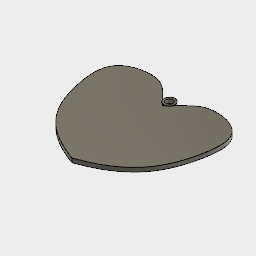
FPROJ_11_LIUYH (Autodesk Fusion 360 design; units mm, degrees)
Autodesk Fusion 360 part; units mm, degrees
sketch "草图1" plane through (0, 0, 0) normal (0, 1, 0) x (1, 0, 0)
  spline S0 degree 5 poles (0, 0) (-0.5793, 0.5821) (-1.7157, 1.7269) (-3.3538, 3.3854) (-5.4045, 5.4793) (-7.7689, 7.8927) (-10.0073, 10.0799) (-12.2674, 11.9974) (-14.7989, 13.5743) (-17.8484, 14.7231) (-21.5675, 15.3505) (-25.8885, 15.3683) (-30.5109, 14.703) (-35.0251, 13.3026) (-39.0061, 11.1441) (-42.1086, 8.2405) (-44.187, 4.6516) (-45.2856, 0.4771) (-45.5576, -4.1594) (-45.2061, -9.1233) (-44.4201, -14.2831) (-43.3041, -19.5247) (-41.886, -24.7523) (-40.1407, -29.8862) (-38.0071, -34.8616) (-35.4076, -39.6274) (-32.2667, -44.1449) (-28.5308, -48.3872) (-24.1657, -52.3367) (-19.1518, -55.9834) (-13.4806, -59.3227) (-8.4167, -61.7474) (-4.3231, -63.4274) (-1.4629, -64.486) (0, -65) knots 0 0 0 0 0 0 0.033333 0.066667 0.1 0.133333 0.166667 0.2 0.233333 0.266667 0.3 0.333333 0.366667 0.4 0.433333 0.466667 0.5 0.533333 0.566667 0.6 0.633333 0.666667 0.7 0.733333 0.766667 0.8 0.833333 0.866667 0.9 0.933333 0.966667 1 1 1 1 1 1
  spline S1 degree 5 poles (0, 0) (0.5793, 0.5821) (1.7157, 1.7269) (3.3538, 3.3854) (5.4045, 5.4793) (7.7689, 7.8927) (10.0073, 10.0799) (12.2674, 11.9974) (14.7989, 13.5743) (17.8484, 14.7231) (21.5675, 15.3505) (25.8885, 15.3683) (30.5109, 14.703) (35.0251, 13.3026) (39.0061, 11.1441) (42.1086, 8.2405) (44.187, 4.6516) (45.2856, 0.4771) (45.5576, -4.1594) (45.2061, -9.1233) (44.4201, -14.2831) (43.3041, -19.5247) (41.886, -24.7523) (40.1407, -29.8862) (38.0071, -34.8616) (35.4076, -39.6274) (32.2667, -44.1449) (28.5308, -48.3872) (24.1657, -52.3367) (19.1518, -55.9834) (13.4806, -59.3227) (8.4167, -61.7474) (4.3231, -63.4274) (1.4629, -64.486) (0, -65) knots 0 0 0 0 0 0 0.033333 0.066667 0.1 0.133333 0.166667 0.2 0.233333 0.266667 0.3 0.333333 0.366667 0.4 0.433333 0.466667 0.5 0.533333 0.566667 0.6 0.633333 0.666667 0.7 0.733333 0.766667 0.8 0.833333 0.866667 0.9 0.933333 0.966667 1 1 1 1 1 1
  point P0 (-10, 10)
  point P1 (-20, 15)
  point P2 (-40, 10)
  point P3 (-45, -10)
  point P4 (-35, -40)
  point P5 (10, 10)
  point P6 (20, 15)
  point P7 (40, 10)
  point P8 (45, -10)
  point P9 (35, -40)
extrude "拉伸1" add sketch "草图1" along normal blind 3 makes body 1
sketch "草图2" plane through (0, 3, 0) normal (0, 1, 0) x (-1, 0, 0)
  spline S0 degree 5 poles (0, 0) (0.5793, -0.5821) (1.7157, -1.7269) (3.3538, -3.3854) (5.4045, -5.4793) (7.7689, -7.8927) (10.0073, -10.0799) (12.2674, -11.9974) (14.7989, -13.5743) (17.8484, -14.7231) (21.5675, -15.3505) (25.8885, -15.3683) (30.5109, -14.703) (35.0251, -13.3026) (39.0061, -11.1441) (42.1086, -8.2405) (44.187, -4.6516) (45.2856, -0.4771) (45.5576, 4.1594) (45.2061, 9.1233) (44.4201, 14.2831) (43.3041, 19.5247) (41.886, 24.7523) (40.1407, 29.8862) (38.0071, 34.8616) (35.4076, 39.6274) (32.2667, 44.1449) (28.5308, 48.3872) (24.1657, 52.3367) (19.1518, 55.9834) (13.4806, 59.3227) (8.4167, 61.7474) (4.3231, 63.4274) (1.4629, 64.486) (0, 65) knots 0 0 0 0 0 0 0.033333 0.066667 0.1 0.133333 0.166667 0.2 0.233333 0.266667 0.3 0.333333 0.366667 0.4 0.433333 0.466667 0.5 0.533333 0.566667 0.6 0.633333 0.666667 0.7 0.733333 0.766667 0.8 0.833333 0.866667 0.9 0.933333 0.966667 1 1 1 1 1 1
  spline S1 degree 5 poles (0, 65) (-1.4629, 64.486) (-4.3231, 63.4274) (-8.4167, 61.7474) (-13.4806, 59.3227) (-19.1518, 55.9834) (-24.1657, 52.3367) (-28.5308, 48.3872) (-32.2667, 44.1449) (-35.4076, 39.6274) (-38.0071, 34.8616) (-40.1407, 29.8862) (-41.886, 24.7523) (-43.3041, 19.5247) (-44.4201, 14.2831) (-45.2061, 9.1233) (-45.5576, 4.1594) (-45.2856, -0.4771) (-44.187, -4.6516) (-42.1086, -8.2405) (-39.0061, -11.1441) (-35.0251, -13.3026) (-30.5109, -14.703) (-25.8885, -15.3683) (-21.5675, -15.3505) (-17.8484, -14.7231) (-14.7989, -13.5743) (-12.2674, -11.9974) (-10.0073, -10.0799) (-7.7689, -7.8927) (-5.4045, -5.4793) (-3.3538, -3.3854) (-1.7157, -1.7269) (-0.5793, -0.5821) (0, 0) knots -1 -1 -1 -1 -1 -1 -0.966667 -0.933333 -0.9 -0.866667 -0.833333 -0.8 -0.766667 -0.733333 -0.7 -0.666667 -0.633333 -0.6 -0.566667 -0.533333 -0.5 -0.466667 -0.433333 -0.4 -0.366667 -0.333333 -0.3 -0.266667 -0.233333 -0.2 -0.166667 -0.133333 -0.1 -0.066667 -0.033333 0 0 0 0 0 0
  circle A0 centre (-75, 0) radius 2.5
  circle A1 centre (-75, 0) radius 4
  dimension "d3" = 5
  dimension "d4" = 8
  measures "d3" diameter of A0
  measures "d4" diameter of A1
extrude "拉伸2" add sketch "草图2" along normal blind 3 separate body contours A1 makes body 2
move_body "移动1" bodies 2 to x (1, 0, 0) y (0, 1, 0) z (0, 0, 1) at (-74.9875, -2.9216, -4.9825)
combine "合并1" operation add target body 1 tool bodies 2
